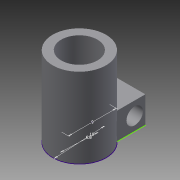
# Autodesk Inventor part: push_clip(2)
Saved by Autodesk Inventor 2015 (Build 190159000, 159)
## iProperties
Created: 2017-10-04
Part Number: push_clip(2)
Material: Generic
Document SubType Name: Modeling
Designer: Anshul
Density: 1 g/cm^3
Appearance: Default
Author: Anshul
Autodesk Inventor part; units mm, degrees
ref_plane "YZ Plane" through (0, 0, 0) normal (1, 0, 0) x (0, 1, 0)
ref_plane "XZ Plane" through (0, 0, 0) normal (0, 1, 0) x (-1, 0, 0)
ref_plane "XY Plane" through (0, 0, 0) normal (0, 0, 1) x (1, 0, 0)
sketch "Sketch1" plane through (0, 0, 0) normal (0, 1, 0) x (-1, 0, 0)
  circle A0 centre (0, 0) radius 3.4
  circle A1 centre (0, 0) radius 5
  line L0 (3.4, 0) -> (3.4, -9)
  line L1 (3.4, -9) -> (-3.4, -9)
  line L2 (-3.4, -9) -> (-3.4, 0)
  dimension "d0" = 6.8
  dimension "d1" = 10
  dimension "d2" = 9
  constraints: 6 end point, 2 centre point, 2 coincident, 2 point on circle, 1 perpendicular, 1 tangent, 1 vertical
  measures "d0" diameter of A0
  measures "d1" diameter of A1
  measures "d2" distance of L0.start L0.end
extrude "Extrusion1" add sketch "Sketch1" along normal blind 5 contours L0 A1 L2 A0 | L0 L1 L2 A1 picked at (2.574, -3.6186)
extrude "Extrusion2" add sketch "Sketch1" along normal blind 15 contours L0 A1 L2 A0 | A0 L2 A1 L0
sketch "Sketch2" plane through (3.4, 0, -9) normal (1, 0, 0) x (0, 0, -1)
  line L0 (0, 5) -> (0, 2.5)
  line L1 (0, 0) -> (0, 5) projected
  line L2 (0, 2.5) -> (-2, 2.5)
  circle A0 centre (-2, 2.5) radius 1.55
  circle A1 centre (-2, 2.5) radius 4
  point P0 (-9, 0)
  dimension "d7" = 2.5
  dimension "d8" = 2
  dimension "d9" = 3.1
  dimension "d10" = 8
  constraints: 4 end point, 2 centre point, 2 coincident, 1 horizontal, 1 midpoint
  measures "d7" distance of L0.start L0.end
  measures "d8" distance of L0.end L2.end
  measures "d9" diameter of A0
  measures "d10" diameter of A1
extrude "Extrusion3" cut sketch "Sketch2" against normal blind 15 contours A0
extrude "Extrusion4" cut sketch "Sketch2" along normal blind 15
sketch "Sketch3" plane through (-3.4, 0, -9) normal (-1, 0, 0) x (0, 0, 1)
  line L0 (0, 5) -> (2, 5)
  line L1 (0, 5) -> (5.3339, 5) projected
  line L2 (2, 5) -> (2, 2.5)
  circle A0 centre (2, 2.5) radius 4
  point P0 (9, 0)
  dimension "d15" = 2
  dimension "d16" = 2.5
  dimension "d17" = 8
  constraints: 4 end point, 1 centre point, 1 coincident, 1 perpendicular, 1 point on line
  measures "d15" distance of L0.start L0.end
  measures "d16" distance of L0.end L2.end
  measures "d17" diameter of A0
extrude "Extrusion5" cut sketch "Sketch3" along normal blind 15
body "Solid1"
